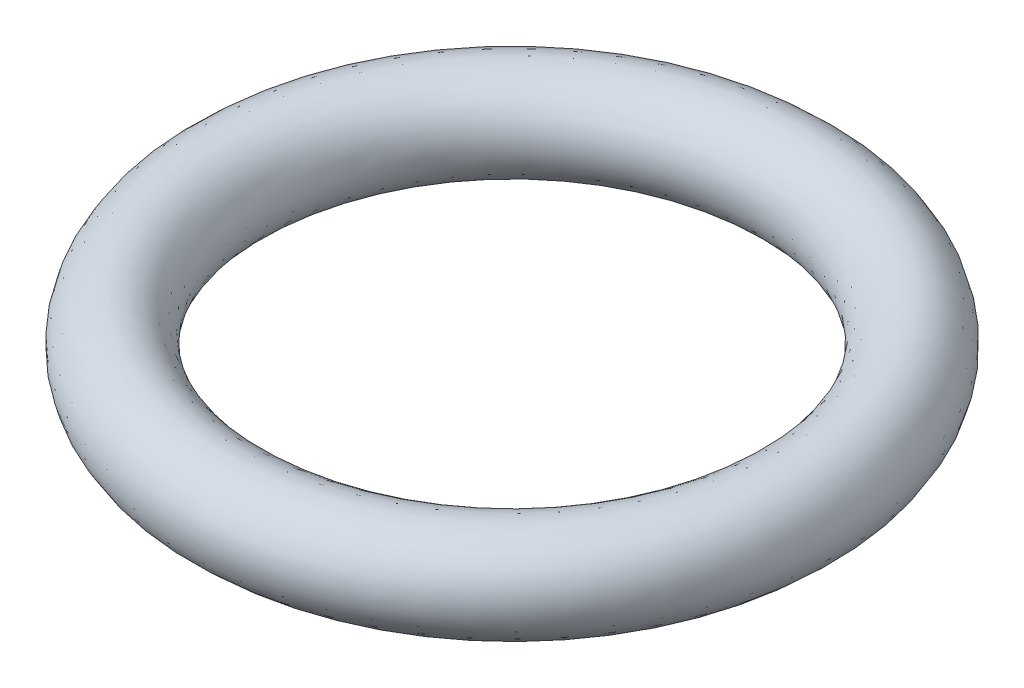
# Autodesk Inventor part: Pulley Ring
Saved by Autodesk Inventor 2023.2 (Build 272271000, 271)
## iProperties
Created: 2023-04-13
Part Number: Pulley Ring
Material: Rubber, Silicone
Document SubType Name: Modeling
Designer: Nathan Cai
Mass: 4.7383 g
Surface Area: 23.878 cm^2
Volume: 3.79064 cm^3
Density: 1.25 g/cm^3
Appearance: Smooth - Dark Forest Green
Author: Nathan Cai
Autodesk Inventor part; units mm, degrees
ref_plane "YZ Plane" through (0, 0, 0) normal (1, 0, 0) x (0, 1, 0)
ref_plane "XZ Plane" through (0, 0, 0) normal (0, 1, 0) x (-1, 0, 0)
ref_plane "XY Plane" through (0, 0, 0) normal (0, 0, 1) x (1, 0, 0)
sketch "Sketch1" plane through (0, 0, 0) normal (1, 0, 0) x (0, 1, 0)
  line L0 (0, 0) -> (0, -19.05) construction
  circle A0 centre (0, -19.05) radius 3.175
  line L1 (0, 0) -> (12.7, 0) construction
  dimension "d0" = 19.05
  dimension "d1" = 6.35
  dimension "d2" = 12.7
  constraints: 4 end point, 1 centre point, 1 coincident, 1 horizontal, 1 vertical
  measures "d0" distance of L0.start L0.end
  measures "d1" diameter of A0
  measures "d2" distance of L0.start L1.end
revolve "Revolution1" add sketch "Sketch1" angle 360 about axis through (0, 0, 0) along (0, 1, 0)
body "Solid1"
